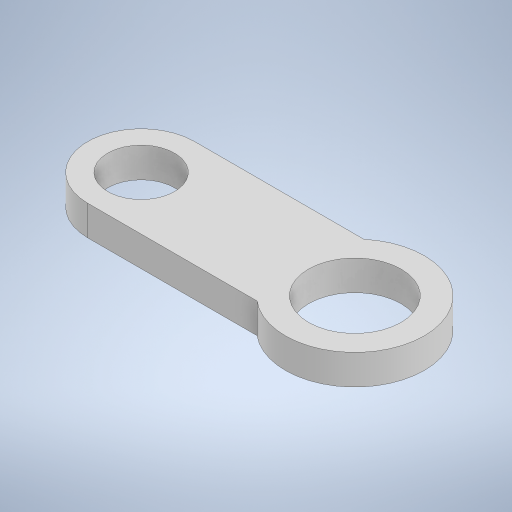
# Autodesk Inventor part: Connecting Rod
Saved by Autodesk Inventor 2023 (Build 270158000, 158)
## iProperties
Created: 2022-10-29
Part Number: Connecting Rod
Material: Generic
Document SubType Name: Modeling
Designer: tommy
Density: 1 g/cm^3
Appearance: Default
Author: tommy
Autodesk Inventor part; units mm, degrees
ref_plane "YZ Plane" through (0, 0, 0) normal (1, 0, 0) x (0, 1, 0)
ref_plane "XZ Plane" through (0, 0, 0) normal (0, 1, 0) x (-1, 0, 0)
ref_plane "XY Plane" through (0, 0, 0) normal (0, 0, 1) x (1, 0, 0)
sketch "Sketch1" plane through (0, 0, 0) normal (0, 1, 0) x (-1, 0, 0)
  arc A0 (19.05, -12.7) -> (19.05, 12.7) centre (19.05, 0) ccw
  arc A1 (-21.2006, 12.7) -> (-21.2006, -12.7) centre (-31.75, 0) ccw
  circle A2 centre (-31.75, 0) radius 10.9982
  circle A3 centre (19.05, 0) radius 7.9375
  line L0 (19.05, -12.7) -> (-24.3756, -12.7)
  line L1 (19.05, 12.7) -> (-24.3756, 12.7)
  line L2 (-31.75, 0) -> (19.05, 0)
  point P0 (0, 0)
  point P1 (-21.2006, 12.7)
  dimension "d4" = 15.875
  dimension "d9" = 50.8
  constraints: 6 end point, 5 point on circle, 4 centre point, 2 coincident, 2 horizontal
  measures "d4" diameter of A3
  measures "d9" distance of L2.start L2.end
extrude "Extrusion1" add sketch "Sketch1" along normal blind 7.1374
body "Solid1"
